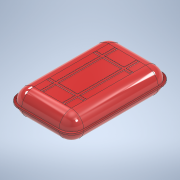
# Autodesk Inventor part: mapContainerPlaceholder
Saved by Autodesk Inventor 2021 (Build 250183000, 183)
## iProperties
Created: 2021-03-02
Part Number: mapContainerPlaceholder
Material: Generic
Document SubType Name: Modeling
Designer: con_c_000
Density: 1 g/cm^3
Appearance: Default
Author: con_c_000
Autodesk Inventor part; units mm, degrees
ref_plane "YZ Plane" through (0, 0, 0) normal (1, 0, 0) x (0, 1, 0)
ref_plane "XZ Plane" through (0, 0, 0) normal (0, 1, 0) x (-1, 0, 0)
ref_plane "XY Plane" through (0, 0, 0) normal (0, 0, 1) x (1, 0, 0)
sketch "Sketch1" plane through (0, 0, 0) normal (0, 0, 1) x (1, 0, 0)
  circle A0 centre (-5.475215, 0) radius 50.8
  circle A1 centre (146.924785, 0) radius 50.8
  line L0 (146.924785, 50.8) -> (-5.475215, 50.8)
  line L1 (-5.475215, -50.8) -> (146.924785, -50.8)
  point P0 (0, 0)
  dimension "d0" = 101.6
  dimension "d1" = 101.6
  dimension "d2" = 152.4
  constraints: 4 end point, 4 point on circle, 3 tangent, 2 centre point
  measures "d0" diameter of A0
  measures "d1" diameter of A1
  measures "d2" distance of A0.centre A1.centre
extrude "Extrusion1" add sketch "Sketch1" along normal blind 406.4
fillet "Fillet1" radius 50.8 4 edges at (-56.2752, 0, 406.4) (70.7248, -50.8, 406.4) (197.7248, 0, 406.4) (70.7248, 50.8, 406.4)
fillet "Fillet2" radius 50.8 4 edges at (-56.2752, 0, 0) (70.7248, -50.8, 0) (197.7248, 0, 0) (70.7248, 50.8, 0)
sketch "Sketch2" plane through (-5.475215, 50.8, 355.6) normal (0, 1, 0) x (1, 0, 0)
  line L0 (-50.8, 0) -> (0, 0) projected
  line L1 (0, 304.8) -> (0, 0) projected
  line L2 (0, 0) -> (0, 304.8)
  line L3 (0, 0) -> (0, 50.8)
  line L4 (0, 50.8) -> (152.4, 50.8)
  line L5 (152.4, 304.8) -> (152.4, 0) projected
  line L6 (152.4, 50.8) -> (152.4, 63.5)
  line L7 (152.4, 63.5) -> (0, 63.5)
  line L8 (0, 304.8) -> (0, 254)
  line L9 (0, 254) -> (152.4, 254)
  line L10 (152.4, 254) -> (152.4, 241.3)
  line L11 (152.4, 241.3) -> (0, 241.3)
  line L12 (152.4, 0) -> (203.2, 0) projected
  line L13 (127, 0) -> (114.3, 0)
  line L14 (114.3, 0) -> (114.3, 304.8)
  line L15 (152.4, 304.8) -> (0, 304.8) projected
  line L16 (127, 0) -> (127, 304.8)
  line L17 (25.4, 0) -> (38.1, 0)
  line L18 (38.1, 0) -> (38.1, 304.8)
  line L19 (25.4, 0) -> (25.4, 304.8)
  line L20 (25.4, 0) -> (38.1, 0)
  line L21 (25.4, 304.8) -> (38.1, 304.8)
  line L22 (114.3, 304.8) -> (127, 304.8)
  point P0 (5.475215, 355.6)
  point P1 (114.3, 63.5)
  point P2 (38.1, 63.5)
  point P3 (38.1, 241.3)
  point P4 (114.3, 241.3)
  point P5 (114.3, 50.8)
  point P6 (127, 50.8)
  point P7 (127, 63.5)
  point P8 (127, 241.3)
  point P9 (127, 254)
  point P10 (114.3, 254)
  point P11 (38.1, 254)
  point P12 (25.4, 254)
  point P13 (0, 241.3)
  point P14 (25.4, 241.3)
  point P15 (25.4, 63.5)
  point P16 (0, 63.5)
  point P17 (0, 50.8)
  point P18 (25.4, 50.8)
  point P19 (38.1, 50.8)
  dimension "d7" = 50.8
  dimension "d8" = 12.7
  dimension "d9" = 50.8
  dimension "d10" = 12.7
  dimension "d11" = 25.4
  dimension "d12" = 12.7
  dimension "d13" = 25.4
  dimension "d14" = 12.7
  constraints: 36 end point, 11 point on line, 8 perpendicular, 4 collinear, 1 parallel
  measures "d7" distance of L0.end L3.end
  measures "d8" distance of L4.end L6.end
  measures "d9" distance of L1.start L8.end
  measures "d10" distance of L9.end L10.end
  measures "d11" distance of L5.end L13.start
  measures "d12" distance of L13.start L13.end
  measures "d13" distance of L0.end L17.start
  measures "d14" distance of L17.start L17.end
extrude "Extrusion2" add sketch "Sketch2" along normal blind 1.27 contours L9 L19 L11 L1 | L15 L18 L9 L19 | L9 L18 L11 L19 | L7 L19 L4 L1 | L11 L18 L7 L19 | L9 L14 L11 L18 | L15 L16 L9 L14 | L7 L18 L4 L19 | L9 L16 L11 L14 | L4 L18 L17 L19 | L7 L14 L4 L18 | L11 L16 L7 L14 | L9 L5 L11 L16 | L7 L16 L4 L14 | L4 L16 L13 L14 | L7 L5 L4 L16
fillet "Fillet3" radius 3.175 1 edges at (32.6248, 52.07, 203.2)
fillet "Fillet4" radius 3.175 31 edges at (121.5248, 52.07, 203.2) (108.8248, 52.07, 203.2) (19.9248, 52.07, 203.2) (32.6248, 52.07, 330.2) (19.9248, 52.07, 330.2) (7.2248, 52.07, 292.1) (7.2248, 52.07, 304.8) (69.4548, 52.07, 292.1) (70.7248, 52.07, 304.8) (134.2248, 52.07, 292.1) (146.9248, 52.07, 298.45) (134.2248, 52.07, 304.8) (121.5248, 52.07, 330.2) (108.8248, 52.07, 330.2) (115.1748, 52.07, 355.6) (146.9248, 52.07, 107.95) (134.2248, 52.07, 101.6) (134.2248, 52.07, 114.3) (108.8248, 52.07, 76.2) (121.5248, 52.07, 76.2) (115.1748, 52.07, 50.8) (70.7248, 52.07, 101.6) (69.4548, 52.07, 114.3) (32.6248, 52.07, 76.2) (19.9248, 52.07, 76.2) (7.2248, 52.07, 101.6) (7.2248, 52.07, 114.3) (-5.4752, 52.07, 107.95) (26.2748, 52.07, 50.8) (26.2748, 52.07, 355.6) (-5.4752, 52.07, 298.45)
sketch "Sketch3" plane through (0, 0, 0) normal (0, 1, 0) x (-1, 0, 0)
  line L0 (62.929571, 412.328113) -> (-203.770429, 412.328113)
  line L1 (-203.770429, 412.328113) -> (-203.770429, -6.771887)
  line L2 (-203.770429, -6.771887) -> (62.929571, -6.771887)
  line L3 (62.929571, -6.771887) -> (62.929571, 412.328113)
  point P0 (0, 0)
  dimension "d19" = 419.1
  dimension "d20" = 266.7
  constraints: 8 end point, 2 parallel, 1 horizontal, 1 perpendicular
  measures "d19" distance between parallel lines of L2 L0
  measures "d20" distance between parallel lines of L3 L1
extrude "Extrusion3" add sketch "Sketch3" along normal mid plane 6.35
fillet "Fillet5" radius 50.8 1 edges at (203.7704, 0, -6.7719)
fillet "Fillet6" radius 50.8 1 edges at (-62.9296, 0, -6.7719)
fillet "Fillet7" radius 50.8 2 edges at (203.7704, 0, 412.3281) (-62.9296, 0, 412.3281)
body "Solid1"
